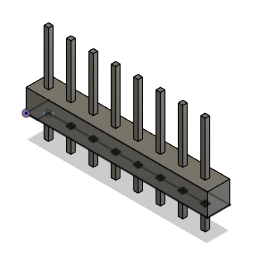
imu_Finger_Holder (Autodesk Fusion 360 archive; units mm, degrees)
design "MPU6050_Headers"
Autodesk Fusion 360 part; units mm, degrees
sketch "Sketch1" plane through (0, 0, 0) normal (0, 1, 0) x (1, 0, 0)
  line L0 (0, 0) -> (20.25, 0)
  line L1 (20.25, 0) -> (20.25, 2.5)
  line L2 (20.25, 2.5) -> (0, 2.5)
  line L3 (0, 2.5) -> (0, 0)
  line L4 (0, 0) -> (1.25, 0)
  line L5 (1.25, 0) -> (1.25, 1.25)
  line L6 (1.5, 1) -> (1, 1)
  line L7 (1, 1) -> (1, 1.5)
  line L8 (1, 1.5) -> (1.5, 1.5)
  line L9 (1.5, 1.5) -> (1.5, 1)
  line L10 (1.5, 1) -> (1, 1.5) construction
  line L11 (1, 1) -> (1.5, 1.5) construction
  line L12 (1.25, 1.25) -> (3.75, 1.25)
  line L13 (4, 1) -> (3.5, 1)
  line L14 (3.5, 1) -> (3.5, 1.5)
  line L15 (3.5, 1.5) -> (4, 1.5)
  line L16 (4, 1.5) -> (4, 1)
  line L17 (4, 1) -> (3.5, 1.5) construction
  line L18 (3.5, 1) -> (4, 1.5) construction
  line L19 (3.75, 1.25) -> (6.25, 1.25)
  line L20 (6.5, 1) -> (6, 1)
  line L21 (6, 1) -> (6, 1.5)
  line L22 (6, 1.5) -> (6.5, 1.5)
  line L23 (6.5, 1.5) -> (6.5, 1)
  line L24 (6.5, 1) -> (6, 1.5) construction
  line L25 (6, 1) -> (6.5, 1.5) construction
  line L26 (6.25, 1.25) -> (8.75, 1.25)
  line L27 (9, 1) -> (8.5, 1)
  line L28 (8.5, 1) -> (8.5, 1.5)
  line L29 (8.5, 1.5) -> (9, 1.5)
  line L30 (9, 1.5) -> (9, 1)
  line L31 (9, 1) -> (8.5, 1.5) construction
  line L32 (8.5, 1) -> (9, 1.5) construction
  line L33 (8.75, 1.25) -> (11.25, 1.25)
  line L34 (11.5, 1.5) -> (11, 1.5)
  line L35 (11, 1.5) -> (11, 1)
  line L36 (11, 1) -> (11.5, 1)
  line L37 (11.5, 1) -> (11.5, 1.5)
  line L38 (11.5, 1.5) -> (11, 1) construction
  line L39 (11, 1.5) -> (11.5, 1) construction
  line L40 (11.25, 1.25) -> (13.75, 1.25)
  line L41 (14, 1.5) -> (13.5, 1.5)
  line L42 (13.5, 1.5) -> (13.5, 1)
  line L43 (13.5, 1) -> (14, 1)
  line L44 (14, 1) -> (14, 1.5)
  line L45 (14, 1.5) -> (13.5, 1) construction
  line L46 (13.5, 1.5) -> (14, 1) construction
  line L47 (13.75, 1.25) -> (16.25, 1.25)
  line L48 (16.5, 1) -> (16, 1)
  line L49 (16, 1) -> (16, 1.5)
  line L50 (16, 1.5) -> (16.5, 1.5)
  line L51 (16.5, 1.5) -> (16.5, 1)
  line L52 (16.5, 1) -> (16, 1.5) construction
  line L53 (16, 1) -> (16.5, 1.5) construction
  line L54 (16.25, 1.25) -> (18.75, 1.25)
  line L55 (19, 1) -> (18.5, 1)
  line L56 (18.5, 1) -> (18.5, 1.5)
  line L57 (18.5, 1.5) -> (19, 1.5)
  line L58 (19, 1.5) -> (19, 1)
  line L59 (19, 1) -> (18.5, 1.5) construction
  line L60 (18.5, 1) -> (19, 1.5) construction
  point P0 (1.25, 1.25)
  point P1 (3.75, 1.25)
  point P2 (6.25, 1.25)
  point P3 (8.75, 1.25)
  point P4 (11.25, 1.25)
  point P5 (13.75, 1.25)
  point P6 (16.25, 1.25)
  point P7 (18.75, 1.25)
  dimension "d1" = 20.25
  dimension "d2" = 0.5
  dimension "d3" = 0.5
  dimension "d4" = 0.5
  dimension "d5" = 0.5
  dimension "d6" = 2.5
  dimension "d7" = 0.5
  dimension "d8" = 0.5
  dimension "d9" = 0.5
  dimension "d10" = 0.5
  dimension "d11" = 2.5
  dimension "d12" = 0.5
  dimension "d13" = 0.5
  dimension "d14" = 2.5
  dimension "d15" = 0.5
  dimension "d16" = 0.5
  dimension "d17" = 2.5
  dimension "d18" = 0.5
  dimension "d19" = 0.5
  dimension "d24" = 2.5
  dimension "d25" = 1.25
  dimension "d26" = 1.25
  dimension "d27" = 2.5
  dimension "d28" = 2.5
  dimension "d29" = 2.5
  constraint horizontal L0
  constraint vertical L1
  constraint horizontal L2
  constraint vertical L3
  constraint coincident L0.start L3.end
  constraint coincident L0 L4.end
  constraint perpendicular L4 L5
  constraint horizontal L6
  constraint perpendicular L6 L7
  constraint parallel L6 L8
  constraint parallel L7 L9
  constraint coincident L10 P0
  constraint coincident L11 P0
  constraint coincident P0 L5.end
  constraint perpendicular L9 L12
  constraint horizontal L13
  constraint perpendicular L13 L14
  constraint parallel L13 L15
  constraint parallel L14 L16
  constraint coincident L17 P1
  constraint coincident L18 P1
  constraint coincident P1 L12.end
  constraint parallel L12 L19
  constraint horizontal L20
  constraint perpendicular L20 L21
  constraint parallel L20 L22
  constraint parallel L21 L23
  constraint coincident L24 P2
  constraint coincident L25 P2
  constraint coincident P2 L19.end
  constraint parallel L19 L26
  constraint horizontal L27
  constraint perpendicular L27 L28
  constraint parallel L27 L29
  constraint parallel L28 L30
  constraint coincident L31 P3
  constraint coincident L32 P3
  constraint coincident P3 L26.end
  constraint parallel L26 L33
  constraint horizontal L34
  constraint perpendicular L34 L35
  constraint parallel L34 L36
  constraint parallel L35 L37
  constraint coincident L38 P4
  constraint coincident L39 P4
  constraint coincident P4 L33.end
  constraint parallel L33 L40
  constraint horizontal L41
  constraint perpendicular L41 L42
  constraint parallel L41 L43
  constraint parallel L42 L44
  constraint coincident L45 P5
  constraint coincident L46 P5
  constraint coincident P5 L40.end
  constraint parallel L40 L47
  constraint horizontal L48
  constraint perpendicular L48 L49
  constraint parallel L48 L50
  constraint parallel L49 L51
  constraint coincident L52 P6
  constraint coincident L53 P6
  constraint coincident P6 L47.end
  constraint parallel L47 L54
  constraint horizontal L55
  constraint perpendicular L55 L56
  constraint parallel L55 L57
  constraint parallel L56 L58
  constraint coincident L59 P7
  constraint coincident L60 P7
  constraint coincident P7 L54.end
  measures "d1" distance of L0.start L0.end
  measures "d2" distance of L14.end L15.end
  measures "d3" distance of L13.end L14.end
  measures "d4" distance of L21.end L22.end
  measures "d5" distance of L20.end L21.end
  measures "d6" distance of P2 P3
  measures "d7" distance of L28.end L29.end
  measures "d8" distance of L27.end L28.end
  measures "d9" distance of L35.end L36.end
  measures "d10" distance of L34.end L35.end
  measures "d11" distance of P4 P5
  measures "d12" distance of L42.end L43.end
  measures "d13" distance of L41.end L42.end
  measures "d14" distance of P5 P6
  measures "d15" distance of L49.end L50.end
  measures "d16" distance of L48.end L49.end
  measures "d17" distance of P6 P7
  measures "d18" distance of L56.end L57.end
  measures "d19" distance of L55.end L56.end
  measures "d24" distance of L0.start L2.end
  measures "d25" distance of L4.end P0
  measures "d26" distance of L0.start L4.end
  measures "d27" distance of P0 P1
  measures "d28" distance of P1 P2
  measures "d29" distance of P3 P4
extrude "Extrude1" add sketch "Sketch1" along normal blind 2.5 makes body 1
extrude "Extrude2" add sketch "Sketch1" along normal blind 8.5 separate body contours L5 L6 L7 L8 L9 L12 | L5 L6 L9 L12 | L12 L14 L15 L16 L19 | L12 L13 L14 L16 L19 | L19 L21 L22 L23 L26 | L19 L20 L21 L23 L26 | L26 L28 L29 L30 L33 | L26 L27 L28 L30 L33 | L33 L34 L35 L37 L40 | L33 L35 L36 L37 L40 | L40 L41 L42 L44 L47 | L40 L42 L43 L44 L47 | L47 L49 L50 L51 L54 | L47 L48 L49 L51 L54 | L55 L56 L57 L58 makes body 2 at (13.6667, 2.8333, -1) makes body 3 at (3.6667, 2.8333, -1.5) makes body 4 at (6, 2.8333, -1.1667) makes body 5 at (16, 2.8333, -1.1667) makes body 6 at (11.1667, 2.8333, -1) makes body 7 at (1.5, 2.8333, -1.3333) makes body 8 at (8.5, 2.8333, -1.1667) makes body 9 at (18.5, 2.8333, -1.1667)
extrude "Extrude3" add sketch "Sketch1" against normal blind 2.5 contours L5 L6 L7 L8 L9 L12 | L5 L6 L9 L12 | L12 L14 L15 L16 L19 | L12 L13 L14 L16 L19 | L19 L21 L22 L23 L26 | L19 L20 L21 L23 L26 | L26 L28 L29 L30 L33 | L26 L27 L28 L30 L33 | L33 L34 L35 L37 L40 | L33 L35 L36 L37 L40 | L40 L41 L42 L44 L47 | L40 L42 L43 L44 L47 | L47 L49 L50 L51 L54 | L47 L48 L49 L51 L54 | L55 L56 L57 L58 bodies 2 1 3 4 5 6 7 8 9
